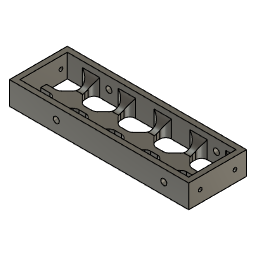
Grill v2 (Autodesk Fusion 360 design; units mm, degrees)
Autodesk Fusion 360 part; units mm, degrees
sketch "Skizze1" plane through (0, 0, 0) normal (0, 0, 1) x (1, 0, 0)
  line L0 (0, 0) -> (155, 0)
  line L1 (155, 0) -> (155, 50)
  line L2 (155, 50) -> (0, 50)
  line L3 (0, 50) -> (0, 0)
  dimension "d1" = 155
  dimension "d2" = 50
  constraint horizontal L0
  constraint vertical L1
  constraint horizontal L2
  constraint vertical L3
  constraint coincident L0.start L3.end
  measures "d1" distance of L0.start L0.end
  measures "d2" distance of L0.start L2.end
extrude "Extrusion1" add sketch "Skizze1" along normal blind 5
sketch "Skizze2" plane through (0, 0, 5) normal (0, 0, 1) x (-1, 0, 0)
  line L0 (0, -50) -> (0, 0)
  line L1 (0, 0) -> (-155, 0)
  line L2 (-155, 0) -> (-155, -50)
  line L3 (-155, -50) -> (0, -50)
  line L4 (-4.5, -45.5) -> (-150.5, -45.5)
  line L5 (-150.5, -45.5) -> (-150.5, -4.5)
  line L6 (-150.5, -4.5) -> (-4.5, -4.5)
  line L7 (-4.5, -4.5) -> (-4.5, -45.5)
  constraint horizontal L4
  constraint vertical L5
  constraint horizontal L6
  constraint vertical L7
extrude "Extrusion2" add sketch "Skizze2" along normal blind 20
sketch "Skizze3" plane through (0, 0, 5) normal (0, 0, 1) x (-1, 0, 0)
  line L0 (-150.5, -4.5) -> (-150.5, -45.5)
  line L1 (-4.5, -45.5) -> (-4.5, -4.5)
  line L2 (-4.5, -22.5) -> (-14.5, -22.5)
  line L3 (-4.5, -27.5) -> (-14.5, -27.5)
  line L4 (-22.5, -45.5) -> (-22.5, -35.5)
  line L5 (-22.5, -4.5) -> (-22.5, -14.5)
  line L6 (-14.5, -22.5) -> (-22.5, -14.5)
  line L7 (-14.5, -27.5) -> (-22.5, -35.5)
  line L8 (-22.5, -4.5) -> (-27.5, -4.5)
  line L9 (-27.5, -45.5) -> (-27.5, -35.5)
  line L10 (-27.5, -4.5) -> (-27.5, -14.5)
  line L11 (-27.5, -4.5) -> (-35.5, -4.5)
  line L12 (-35.5, -4.5) -> (-35.5, -22.5)
  line L13 (-27.5, -35.5) -> (-35.5, -27.5)
  line L14 (-27.5, -14.5) -> (-35.5, -22.5)
  line L15 (-35.5, -22.5) -> (-45.5, -22.5)
  line L16 (-35.5, -27.5) -> (-45.5, -27.5)
  line L17 (-35.5, -4.5) -> (-53.5, -4.5)
  line L18 (-53.5, -4.5) -> (-53.5, -14.5)
  line L19 (-45.5, -22.5) -> (-53.5, -14.5)
  line L20 (-53.5, -45.5) -> (-53.5, -35.5)
  line L21 (-53.5, -35.5) -> (-45.5, -27.5)
  line L22 (-53.5, -45.5) -> (-58.5, -45.5)
  line L23 (-58.5, -45.5) -> (-58.5, -35.5)
  line L24 (-53.5, -4.5) -> (-58.5, -4.5)
  line L25 (-58.5, -4.5) -> (-58.5, -14.5)
  line L26 (-58.5, -4.5) -> (-66.5, -4.5)
  line L27 (-66.5, -4.5) -> (-66.5, -22.5)
  line L28 (-58.5, -14.5) -> (-66.5, -22.5)
  line L29 (-66.5, -27.5) -> (-58.5, -35.5)
  line L30 (-66.5, -27.5) -> (-76.5, -27.5)
  line L31 (-66.5, -22.5) -> (-76.5, -22.5)
  line L32 (-76.5, -4.5) -> (-84.5, -4.5)
  line L33 (-84.5, -4.5) -> (-84.5, -14.5)
  line L34 (-84.5, -14.5) -> (-76.5, -22.5)
  line L35 (-76.5, -27.5) -> (-84.5, -35.5)
  line L36 (-84.5, -35.5) -> (-84.5, -45.5)
  line L37 (-84.5, -45.5) -> (-89.5, -45.5)
  line L38 (-89.5, -45.5) -> (-89.5, -35.5)
  line L39 (-89.5, -35.5) -> (-97.5, -27.5)
  line L40 (-89.5, -35.5) -> (-78.1863, -35.5) construction
  line L41 (-97.5, -27.5) -> (-107.5, -27.5)
  line L42 (-107.5, -27.5) -> (-115.5, -35.5)
  line L43 (-115.5, -35.5) -> (-115.5, -45.5)
  line L44 (-84.5, -4.5) -> (-89.5, -4.5)
  line L45 (-89.5, -4.5) -> (-89.5, -14.5)
  line L46 (-89.5, -14.5) -> (-97.5, -22.5)
  line L47 (-89.5, -14.5) -> (-78.1863, -14.5) construction
  line L48 (-97.5, -22.5) -> (-107.5, -22.5)
  line L49 (-107.5, -22.5) -> (-115.5, -14.5)
  line L50 (-115.5, -14.5) -> (-115.5, -4.5)
  line L51 (-115.5, -4.5) -> (-120.5, -4.5)
  line L52 (-120.5, -4.5) -> (-120.5, -14.5)
  line L53 (-120.5, -14.5) -> (-128.5, -22.5)
  line L54 (-120.5, -14.5) -> (-109.1863, -14.5) construction
  line L55 (-128.5, -22.5) -> (-138.5, -22.5)
  line L56 (-138.5, -22.5) -> (-146.5, -14.5)
  line L57 (-138.5, -22.5) -> (-127.1863, -22.5) construction
  line L58 (-146.5, -14.5) -> (-146.5, -4.5)
  line L59 (-138.5, -27.5) -> (-146.5, -35.5)
  line L60 (-146.5, -35.5) -> (-146.5, -45.5)
  line L61 (-138.5, -27.5) -> (-128.5, -27.5)
  line L62 (-128.5, -27.5) -> (-120.5, -35.5)
  line L63 (-128.5, -27.5) -> (-117.1863, -27.5) construction
  line L64 (-120.5, -35.5) -> (-120.5, -45.5)
  line L65 (-4.5, -27.5) -> (-4.5, -45.5)
  line L66 (-4.5, -45.5) -> (-22.5, -45.5)
  line L67 (-4.5, -22.5) -> (-4.5, -4.5)
  line L68 (-4.5, -4.5) -> (-22.5, -4.5)
  line L69 (-27.5, -4.5) -> (-53.5, -4.5)
  line L70 (-58.5, -4.5) -> (-84.5, -4.5)
  line L71 (-89.5, -4.5) -> (-115.5, -4.5)
  line L72 (-120.5, -4.5) -> (-146.5, -4.5)
  line L73 (-146.5, -45.5) -> (-120.5, -45.5)
  line L74 (-115.5, -45.5) -> (-89.5, -45.5)
  line L75 (-84.5, -45.5) -> (-58.5, -45.5)
  line L76 (-53.5, -45.5) -> (-27.5, -45.5)
  dimension "d13" = 10
  dimension "d14" = 10
  dimension "d15" = 18
  dimension "d16" = 10
  dimension "d17" = 18
  dimension "d18" = 10
  dimension "d19" = 5
  dimension "d20" = 5
  dimension "d21" = 10
  dimension "d22" = 10
  dimension "d23" = 8
  dimension "d24" = 18
  dimension "d25" = 5
  dimension "d26" = 10
  dimension "d27" = 10
  dimension "d28" = 18
  dimension "d29" = 10
  dimension "d30" = 10
  dimension "d31" = 5
  dimension "d32" = 10
  dimension "d33" = 5
  dimension "d34" = 10
  dimension "d35" = 8
  dimension "d36" = 18
  dimension "d37" = 5
  dimension "d38" = 10
  dimension "d39" = 10
  dimension "d40" = 8
  dimension "d41" = 10
  dimension "d42" = 5
  dimension "d43" = 10
  dimension "d44" = 135
  dimension "d45" = 10
  dimension "d46" = 5
  dimension "d47" = 10
  dimension "d48" = 135
  dimension "d49" = 10
  dimension "d50" = 5
  dimension "d51" = 10
  dimension "d52" = 135
  dimension "d53" = 10
  dimension "d54" = 135
  dimension "d56" = 10
  dimension "d57" = 45
  constraint perpendicular L1 L3
  constraint perpendicular L5 L8
  constraint perpendicular L8 L10
  constraint perpendicular L10 L11
  constraint perpendicular L11 L12
  constraint perpendicular L12 L17
  constraint perpendicular L17 L18
  constraint perpendicular L20 L22
  constraint perpendicular L18 L24
  constraint perpendicular L24 L25
  constraint perpendicular L25 L26
  constraint perpendicular L26 L27
  constraint perpendicular L28 L29
  constraint perpendicular L27 L31
  constraint perpendicular L32 L33
  constraint perpendicular L34 L35
  constraint perpendicular L36 L37
  constraint perpendicular L37 L38
  constraint horizontal L40
  constraint perpendicular L38 L41
  constraint perpendicular L39 L42
  constraint perpendicular L33 L44
  constraint perpendicular L44 L45
  constraint horizontal L47
  constraint perpendicular L46 L49
  constraint perpendicular L50 L51
  constraint horizontal L54
  constraint horizontal L57
  constraint horizontal L63
  constraint coincident L1.start L65.end
  constraint perpendicular L3 L65
  constraint perpendicular L65 L66
  constraint coincident L1.end L67.end
  constraint perpendicular L2 L67
  constraint perpendicular L5 L68
  constraint perpendicular L33 L70
  constraint perpendicular L50 L71
  constraint perpendicular L58 L72
  constraint perpendicular L64 L73
  constraint perpendicular L38 L74
  constraint perpendicular L23 L75
  constraint perpendicular L9 L76
  measures "d13" distance of L2.start L2.end
  measures "d14" distance of L3.start L3.end
  measures "d15" distance of L1.start L4.start
  measures "d16" distance of L4.start L4.end
  measures "d17" distance of L1.end L5.start
  measures "d18" distance of L5.start L5.end
  measures "d19" distance of L4.start L9.start
  measures "d20" distance of L5.start L8.end
  measures "d21" distance of L9.start L9.end
  measures "d22" distance of L8.end L10.end
  measures "d23" distance of L8.end L11.end
  measures "d24" distance of L11.end L12.end
  measures "d25" distance of L12.end L13.end
  measures "d26" distance of L12.end L15.end
  measures "d27" distance of L13.end L16.end
  measures "d28" distance of L11.end L17.end
  measures "d29" distance of L17.end L18.end
  measures "d30" distance of L20.start L20.end
  measures "d31" distance of L20.start L22.end
  measures "d32" distance of L22.end L23.end
  measures "d33" distance of L17.end L24.end
  measures "d34" distance of L24.end L25.end
  measures "d35" distance of L24.end L26.end
  measures "d36" distance of L26.end L27.end
  measures "d37" distance of L27.end L29.start
  measures "d38" distance of L29.start L30.end
  measures "d39" distance of L27.end L31.end
  measures "d40" distance of L32.start L32.end
  measures "d41" distance of L32.end L33.end
  measures "d42" distance of L36.end L37.end
  measures "d43" distance of L37.end L38.end
  measures "d44" angle of L39 L40
  measures "d45" distance of L39.end L41.end
  measures "d46" distance of L32.end L44.end
  measures "d47" distance of L44.end L45.end
  measures "d48" angle of L46 L47
  measures "d49" distance of L46.end L48.end
  measures "d50" distance of L50.end L51.end
  measures "d51" distance of L51.end L52.end
  measures "d52" angle of L53 L54
  measures "d53" distance of L53.end L55.end
  measures "d54" angle of L56 L57
  measures "d56" distance of L59.start L61.end
  measures "d57" angle of L62 L63
extrude "Extrusion3" cut sketch "Skizze3" against normal blind 5
fillet "Abrundung1" radius 5 56 edges at (22.5, 45.5, 2.5) (53.5, 45.5, 2.5) (84.5, 45.5, 2.5) (115.5, 45.5, 2.5) (146.5, 45.5, 2.5) (146.5, 35.5, 2.5) (120.5, 35.5, 2.5) (128.5, 27.5, 2.5) (138.5, 27.5, 2.5) (115.5, 35.5, 2.5) (107.5, 27.5, 2.5) (97.5, 27.5, 2.5) (89.5, 35.5, 2.5) (89.5, 45.5, 2.5) (120.5, 45.5, 2.5) (146.5, 14.5, 2.5) (138.5, 22.5, 2.5) (128.5, 22.5, 2.5) (120.5, 14.5, 2.5) (115.5, 14.5, 2.5) (107.5, 22.5, 2.5) (97.5, 22.5, 2.5) (89.5, 14.5, 2.5) (84.5, 35.5, 2.5) (84.5, 14.5, 2.5) (76.5, 22.5, 2.5) (76.5, 27.5, 2.5) (66.5, 27.5, 2.5) (66.5, 22.5, 2.5) (58.5, 14.5, 2.5) (58.5, 35.5, 2.5) (58.5, 45.5, 2.5) (53.5, 35.5, 2.5) (45.5, 27.5, 2.5) (45.5, 22.5, 2.5) (53.5, 14.5, 2.5) (35.5, 27.5, 2.5) (35.5, 22.5, 2.5) (27.5, 14.5, 2.5) (27.5, 35.5, 2.5) (27.5, 45.5, 2.5) (22.5, 35.5, 2.5) (14.5, 27.5, 2.5) (14.5, 22.5, 2.5) (22.5, 14.5, 2.5) (146.5, 4.5, 2.5) (120.5, 4.5, 2.5) (115.5, 4.5, 2.5) (84.5, 4.5, 2.5) (89.5, 4.5, 2.5) (58.5, 4.5, 2.5) (53.5, 4.5, 2.5) (27.5, 4.5, 2.5) (22.5, 4.5, 2.5) (4.5, 22.5, 2.5) (4.5, 27.5, 2.5)
fillet "Abrundung2" radius 10 5 edges at (25, 45.5, 5) (56, 45.5, 5) (87, 45.5, 5) (118, 45.5, 5) (146, 45.5, 5)
fillet "Abrundung3" radius 10 5 edges at (146, 4.5, 5) (118, 4.5, 5) (87, 4.5, 5) (56, 4.5, 5) (25, 4.5, 5)
extrude "Extrusion4" cut 1 faces at (53.1667, 48.5, 25) along direction (0, 0, -1) blind 5
hole "Bohrung1" at (0, 40, 10) direction (1, 0, 0) diameter 3.2 depth 10 tip angle 180
hole "Bohrung2" at (0, 10, 10) direction (1, 0, 0) diameter 3.2 depth 10 tip angle 180
hole "Bohrung3" at (40.5, 45.5, 10) direction (0, 1, 0) diameter 5.2 depth 10 tip angle 180
hole "Bohrung4" at (133.5, 45.5, 10) direction (0, 1, 0) diameter 5.2 depth 10 tip angle 180
hole "Bohrung5" at (133.5, 4.5, 10) direction (0, -1, 0) diameter 5.2 depth 10 tip angle 180
hole "Bohrung6" at (40.5, 4.5, 10) direction (0, -1, 0) diameter 5.2 depth 10 tip angle 180
delete_face "Fläche löschen1" 1 faces at (9.2621, 27.5057, 3.3333)
delete_face "Fläche löschen2" 1 faces at (9.2621, 22.4943, 3.3333)
hole "Bohrung7" at (155, 40, 10) direction (-1, 0, 0) diameter 3.2 depth 10 tip angle 180
hole "Bohrung8" at (155, 10, 10) direction (-1, 0, 0) diameter 3.2 depth 10 tip angle 180
